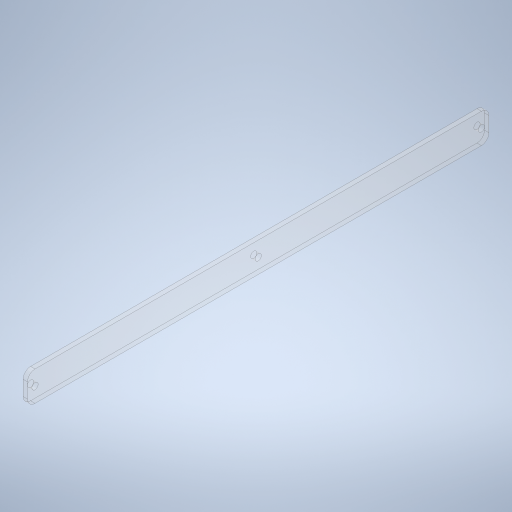
# Autodesk Inventor part: x바
Saved by Autodesk Inventor 2024 (Build 280153000, 153)
## iProperties
Created: 2024-04-11
Part Number: x바
Material: PMMA 플라스틱
Document SubType Name: Modeling
Designer: kkamin5
Density: 1.188 g/cm^3
Appearance: 폴리카보네이트 - 선명
Author: kkamin5
Autodesk Inventor part; units mm, degrees
ref_plane "YZ Plane" through (0, 0, 0) normal (1, 0, 0) x (0, 1, 0)
ref_plane "XZ Plane" through (0, 0, 0) normal (0, 1, 0) x (-1, 0, 0)
ref_plane "XY Plane" through (0, 0, 0) normal (0, 0, 1) x (1, 0, 0)
sketch "스케치1" plane through (0, 0, 0) normal (1, 0, 0) x (0, 1, 0)
  line L0 (10, 155) -> (-10, 155)
  line L1 (-10, 155) -> (-10, -155)
  line L2 (-10, -155) -> (10, -155)
  line L3 (10, -155) -> (10, 155)
  point P0 (0, 0)
  dimension "d0" = 20
  dimension "d1" = 310
  dimension "d2" = 155
  dimension "d3" = 10
  constraints: 8 end point, 2 parallel, 1 horizontal, 1 perpendicular
  measures "d0" distance of L2.end L1.end
  measures "d1" distance of L1.end L0.end
  measures "d2" distance from line of point (0, 0) L0
  measures "d3" distance from line of point (0, 0) L3
extrude "돌출1" add sketch "스케치1" along normal blind 3
sketch "스케치2" plane through (3, 0, 0) normal (1, 0, 0) x (0, 0, -1)
  line L0 (155, -10) -> (155, 10) construction
  line L1 (-155, -10) -> (155, -10) construction
  line L2 (155, 10) -> (-155, 10) construction
  line L3 (-155, 10) -> (-155, -10) construction
  line L4 (-155, -10) -> (155, -10) construction
  line L5 (155, -10) -> (155, 10) construction
  circle A0 centre (-150, 0) radius 10
  line L6 (0, 30.1702) -> (0, -32.7661) construction
  circle A1 centre (150, 0) radius 10
  dimension "d6" = 5
  dimension "d7" = 10
  dimension "d8" = 5
  dimension "d9" = 10
  constraints: 10 end point, 2 centre point, 2 coincident, 2 parallel, 2 tangent, 1 horizontal, 1 perpendicular, 1 vertical
  measures "d6" distance from line of L3 A0.centre
  measures "d7" distance from line of L1 A0.centre
  measures "d8" distance from line of L0 A1.centre
  measures "d9" distance from line of L1 A1.centre
hole "구멍1" at (3, 0, -150) at (3, 0, 150) direction (-1, 0, 0) diameter 4.2 end through all
fillet "모깎기1" radius 5 4 edges at (1.5, 10, 155) (1.5, -10, 155) (1.5, -10, -155) (1.5, 10, -155)
sketch "스케치3" plane through (3, 0, 0) normal (1, 0, 0) x (0, 0, -1)
  circle A0 centre (0, 0) radius 2.1
  dimension "d18" = 4.2
  constraints: 1 centre point, 1 coincident
  measures "d18" diameter of A0
extrude "돌출2" cut sketch "스케치3" against normal through all
equation "\"d2\" = 0.5 * d1"
equation "\"d3\" = 0.5 * d0"
